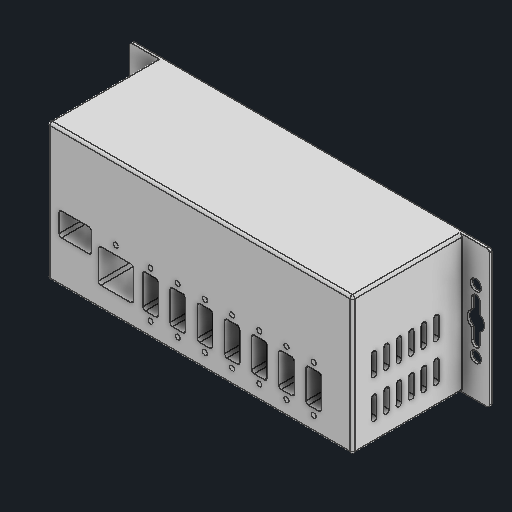
# Autodesk Inventor part: StarTech7PortUSB3Hub
Saved by Autodesk Inventor 2025.2 (Build 292293000, 293)
## iProperties
Created: 2025-10-31
Part Number: StarTech7PortUSB3Hub
Material: Generic
Document SubType Name: Modeling
Designer: valer
Density: 1 g/cm^3
Appearance: Default
Author: valer
Autodesk Inventor part; units mm, degrees
ref_plane "YZ Plane" through (0, 0, 0) normal (1, 0, 0) x (0, 1, 0)
ref_plane "XZ Plane" through (0, 0, 0) normal (0, 1, 0) x (-1, 0, 0)
ref_plane "XY Plane" through (0, 0, 0) normal (0, 0, 1) x (1, 0, 0)
sketch "Base" plane through (0, 0, 0) normal (0, 0, 1) x (1, 0, 0)
  line L0 (-72.25, -27.5) -> (72.25, -27.5)
  line L1 (72.25, -27.5) -> (72.25, 27.5)
  line L2 (72.25, 27.5) -> (-72.25, 27.5)
  line L3 (-72.25, 27.5) -> (-72.25, -27.5)
  line L4 (-72.25, -27.5) -> (72.25, 27.5) construction
  line L5 (72.25, -27.5) -> (-72.25, 27.5) construction
  line L6 (-66.75, 27.5) -> (-66.75, -27.5) construction
  line L7 (-101.15, 0) -> (101.15, 0) construction
  line L8 (0, -38.5) -> (0, 38.5) construction
  line L9 (66.75, 27.5) -> (66.75, -27.5) construction
  circle A0 centre (-66.75, 12.5) radius 2.25
  circle A1 centre (-66.75, -12.5) radius 2.25
  circle A2 centre (66.75, 12.5) radius 2.25
  circle A3 centre (66.75, -12.5) radius 2.25
  circle A4 centre (-66.75, 0) radius 3.5
  circle A5 centre (66.75, 0) radius 3.5
  circle A6 centre (-66.75, 7.5) radius 1.75
  circle A7 centre (-66.75, -7.5) radius 1.75
  line L10 (-68.5, 7.5) -> (-68.5, -7.5)
  line L11 (-65, 7.5) -> (-65, -7.5)
  circle A8 centre (66.75, 7.5) radius 1.75
  circle A9 centre (66.75, -7.5) radius 1.75
  line L12 (68.5, 7.5) -> (68.5, -7.5)
  line L13 (65, 7.5) -> (65, -7.5)
  point P0 (0, 0)
  point P1 (-65, -3.0311)
  point P2 (-68.5, -3.0311)
  point P3 (-68.5, 3.0311)
  point P4 (-65, 3.0311)
  point P5 (65, -3.0311)
  point P6 (65, 3.0311)
  point P7 (68.5, 3.0311)
  point P8 (68.5, -3.0311)
  dimension "d0" = 144.5
  dimension "d1" = 55
  dimension "d2" = 133.5
  dimension "d3" = 4.5
  dimension "d4" = 15
  dimension "d5" = 7
  dimension "d6" = 3.5
  dimension "d7" = 20
  constraints: 24 end point, 13 symmetric about line, 10 centre point, 8 point on circle, 5 point on line, 4 tangent, 3 midpoint, 2 parallel, 2 perpendicular, 1 horizontal, 7 other
  measures "d0" distance of L1.end L2.end
  measures "d1" distance of L0.end L1.end
  measures "d2" distance between parallel lines of L9 L6
  measures "d3" diameter of A0
  measures "d4" distance from line of L2 A0.centre
  measures "d5" diameter of A4
  measures "d6" diameter of A6
  measures "d7" distance of A1.centre A6.centre
extrude "BaseFeature" add sketch "Base" along normal blind 1
fillet "BaseFilletsFeature" radius 1 4 edges at (-72.25, -27.5, 0.5) (-72.25, 27.5, 0.5) (72.25, -27.5, 0.5) (72.25, 27.5, 0.5)
sketch "Sketch2" plane through (0, 0, 1) normal (0, 0, 1) x (1, 0, 0)
  line L0 (71.25, 27.5) -> (-71.25, 27.5) projected
  line L1 (-71.25, -27.5) -> (71.25, -27.5) projected
  line L2 (-61.25, 27.5) -> (61.25, 27.5)
  line L3 (61.25, 27.5) -> (61.25, -27.5)
  line L4 (61.25, -27.5) -> (-61.25, -27.5)
  line L5 (-61.25, -27.5) -> (-61.25, 27.5)
  line L6 (-72.25, 26.5) -> (-72.25, -26.5) projected
  line L7 (72.25, -26.5) -> (72.25, 26.5) projected
  point P0 (0, 0)
  point P1 (-61.25, -27.5)
  point P2 (61.25, 27.5)
  dimension "d11" = 11
  dimension "d12" = 11
  constraints: 8 end point, 2 parallel, 2 point on line, 1 horizontal, 1 perpendicular
  measures "d11" distance between parallel lines of L6 L5
  measures "d12" distance between parallel lines of L7 L3
extrude "BodyFeature" add sketch "Sketch2" along normal blind 44
fillet "BodyFilletsFeature" radius 1 4 edges at (-61.25, -27.5, 23) (-61.25, 27.5, 23) (61.25, -27.5, 23) (61.25, 27.5, 23)
sketch "Sketch3" plane through (0, 0, 45) normal (0, 0, 1) x (1, 0, 0)
  line L0 (-40.8, -1.85) -> (48.77, -1.85) construction
  line L1 (48.77, -1.85) -> (48.77, -22.35) construction
  line L2 (48.77, -22.35) -> (-40.8, -22.35) construction
  line L3 (-40.8, -22.35) -> (-40.8, -1.85) construction
  arc A0 (65, 3.0311) -> (65, -3.0311) centre (66.75, 0) ccw projected
  line L4 (48.77, -2.85) -> (-40.8, -2.85) construction
  line L5 (48.77, -12.1) -> (-40.8, -12.1) construction
  circle A1 centre (45.67, -2.85) radius 1
  line L6 (42.57, -5.35) -> (48.77, -5.35)
  line L7 (48.77, -5.35) -> (48.77, -18.85)
  line L8 (48.77, -18.85) -> (42.57, -18.85)
  line L9 (42.57, -18.85) -> (42.57, -5.35)
  line L10 (45.67, -2.85) -> (45.67, -12.1) construction
  circle A2 centre (45.67, -21.35) radius 1
  line L11 (61.25, -26.5) -> (61.25, 26.5) construction
  line L12 (31.65, -5.35) -> (37.85, -5.35)
  line L13 (31.65, -18.85) -> (31.65, -5.35)
  line L14 (37.85, -18.85) -> (31.65, -18.85)
  line L15 (37.85, -5.35) -> (37.85, -18.85)
  circle A3 centre (34.75, -2.85) radius 1
  circle A4 centre (34.75, -21.35) radius 1
  line L16 (20.73, -5.35) -> (26.93, -5.35)
  line L17 (20.73, -18.85) -> (20.73, -5.35)
  line L18 (26.93, -18.85) -> (20.73, -18.85)
  line L19 (26.93, -5.35) -> (26.93, -18.85)
  circle A5 centre (23.83, -2.85) radius 1
  circle A6 centre (23.83, -21.35) radius 1
  line L20 (9.81, -5.35) -> (16.01, -5.35)
  line L21 (9.81, -18.85) -> (9.81, -5.35)
  line L22 (16.01, -18.85) -> (9.81, -18.85)
  line L23 (16.01, -5.35) -> (16.01, -18.85)
  circle A7 centre (12.91, -2.85) radius 1
  circle A8 centre (12.91, -21.35) radius 1
  line L24 (-1.11, -5.35) -> (5.09, -5.35)
  line L25 (-1.11, -18.85) -> (-1.11, -5.35)
  line L26 (5.09, -18.85) -> (-1.11, -18.85)
  line L27 (5.09, -5.35) -> (5.09, -18.85)
  circle A9 centre (1.99, -2.85) radius 1
  circle A10 centre (1.99, -21.35) radius 1
  line L28 (-12.03, -5.35) -> (-5.83, -5.35)
  line L29 (-12.03, -18.85) -> (-12.03, -5.35)
  line L30 (-5.83, -18.85) -> (-12.03, -18.85)
  line L31 (-5.83, -5.35) -> (-5.83, -18.85)
  circle A11 centre (-8.93, -2.85) radius 1
  circle A12 centre (-8.93, -21.35) radius 1
  line L32 (-22.95, -5.35) -> (-16.75, -5.35)
  line L33 (-22.95, -18.85) -> (-22.95, -5.35)
  line L34 (-16.75, -18.85) -> (-22.95, -18.85)
  line L35 (-16.75, -5.35) -> (-16.75, -18.85)
  circle A13 centre (-19.85, -2.85) radius 1
  circle A14 centre (-19.85, -21.35) radius 1
  line L36 (-26.8, -5.35) -> (-40.8, -5.35)
  line L37 (-40.8, -5.35) -> (-40.8, -18.85)
  line L38 (-40.8, -18.85) -> (-26.8, -18.85)
  line L39 (-26.8, -18.85) -> (-26.8, -5.35)
  line L40 (-33.8, -2.85) -> (-33.8, -22.35) construction
  line L41 (-56.6, -0.85) -> (-43.6, -0.85)
  line L42 (-43.6, -0.85) -> (-43.6, -10.25)
  line L43 (-43.6, -10.25) -> (-56.6, -10.25)
  line L44 (-56.6, -10.25) -> (-56.6, -0.85)
  line L45 (-61.25, 26.5) -> (-61.25, -26.5) construction
  circle A15 centre (-33.8, -1.85) radius 1
  circle A16 centre (-33.8, -22.35) radius 1
  circle A17 centre (-45.1, -13.6) radius 1.5
  line L46 (-43.6, -10.25) -> (-43.6, -13.6) construction
  line L47 (-40.8, -12.1) -> (-45.1, -12.1) construction
  point P0 (0, 0)
  point P1 (42.57, -12.1)
  point P2 (45.67, -5.35)
  point P3 (34.75, -5.35)
  point P4 (31.65, -12.1)
  point P5 (23.83, -5.35)
  point P6 (20.73, -12.1)
  point P7 (12.91, -5.35)
  point P8 (9.81, -12.1)
  point P9 (1.99, -5.35)
  point P10 (-1.11, -12.1)
  point P11 (-8.93, -5.35)
  point P12 (-12.03, -12.1)
  point P13 (-19.85, -5.35)
  point P14 (-22.95, -12.1)
  point P15 (-33.8, -5.35)
  point P16 (-50.1, -10.25)
  point P17 (-26.8, -12.1)
  dimension "d16" = 12.1
  dimension "d17" = 2
  dimension "d18" = 13.5
  dimension "d19" = 6.2
  dimension "d20" = 18.5
  dimension "d21" = 12.48
  dimension "d24" = 10.92
  dimension "d29" = 14
  dimension "d30" = 13.95
  dimension "d31" = 16.3
  dimension "d32" = 9.4
  dimension "d33" = 11.15
  dimension "d34" = 1
  dimension "d35" = 13
  dimension "d36" = 3
  constraints: 92 end point, 17 centre point, 12 point on line, 9 parallel, 7 midpoint, 7 perpendicular, 5 horizontal, 4 collinear, 3 tangent, 2 equal radius, 2 point on circle, 1 coincident, 1 symmetric about line, 85 other
  measures "d16" vertical distance of A0.centre L5.start
  measures "d17" diameter of A1
  measures "d18" distance of L6.end L7.end
  measures "d19" distance between parallel lines of L9 L7
  measures "d20" distance from line of A2.centre L4
  measures "d21" distance between parallel lines of L11 L1
  measures "d24" distance of L6.start L12.start
  measures "d29" distance of L37.end L38.end
  measures "d30" distance from line of A14.centre L40
  measures "d31" distance from line of point (-50.1, -10.25) L40
  measures "d32" distance of L41.end L42.end
  measures "d33" distance from line of L45 point (-50.1, -10.25)
  measures "d34" distance between parallel lines of L0 L41
  measures "d35" distance of L42.end L43.end
  measures "d36" diameter of A17
extrude "PortsFeature" cut sketch "Sketch3" against normal blind 20 contours A1 | L6 L7 L8 L9 | A2 | L12 L15 L14 L13 | A3 | A4 | L16 L19 L18 L17 | A5 | A6 | L20 L23 L22 L21 | A7 | A8 | L24 L27 L26 L25 | A9 | A10 | L28 L31 L30 L29 | A11 | A12 | L32 L35 L34 L33 | A13 | A14 | L39 L38 L37 L36 | L41 L42 L43 L44 | A15
fillet "PortFilletsFeature" radius 1 36 edges at (48.77, -5.35, 35) (42.57, -5.35, 35) (42.57, -18.85, 35) (48.77, -18.85, 35) (37.85, -5.35, 35) (31.65, -5.35, 35) (31.65, -18.85, 35) (37.85, -18.85, 35) (26.93, -5.35, 35) (20.73, -5.35, 35) (20.73, -18.85, 35) (26.93, -18.85, 35) (16.01, -5.35, 35) (9.81, -5.35, 35) (9.81, -18.85, 35) (16.01, -18.85, 35) (5.09, -5.35, 35) (-1.11, -5.35, 35) (-1.11, -18.85, 35) (5.09, -18.85, 35) (-5.83, -5.35, 35) (-12.03, -5.35, 35) (-12.03, -18.85, 35) (-5.83, -18.85, 35) (-16.75, -5.35, 35) (-22.95, -5.35, 35) (-22.95, -18.85, 35) (-16.75, -18.85, 35) (-26.8, -5.35, 35) (-40.8, -5.35, 35) (-40.8, -18.85, 35) (-26.8, -18.85, 35) (-43.6, -0.85, 35) (-56.6, -0.85, 35) (-56.6, -10.25, 35) (-43.6, -10.25, 35)
fillet "OutsideFilletsFeature" radius 1 8 edges at (-60.9571, 27.2071, 45) (-61.25, 0, 45) (-60.9571, -27.2071, 45) (0, -27.5, 45) (60.9571, -27.2071, 45) (61.25, 0, 45) (60.9571, 27.2071, 45) (0, 27.5, 45)
sketch "Sketch4" plane through (61.25, -26.5, 1) normal (1, 0, 0) x (0, 0, -1)
  line L0 (-44, 7.65) -> (-24, 7.65) construction
  line L1 (-35.35, 7.65) -> (0, 7.65) construction
  line L2 (0, 7.65) -> (0, 15.65) construction
  line L3 (0, 15.65) -> (-35.35, 15.65) construction
  line L4 (-35.35, 15.65) -> (-35.35, 7.65) construction
  line L5 (-43, -1) -> (0, -1) projected
  line L6 (-44, 53) -> (-44, 0) projected
  line L7 (-35.35, 22.85) -> (-35.35, 14.85) construction
  line L8 (-35.35, 14.85) -> (0, 14.85) construction
  line L9 (0, 22.85) -> (-35.35, 22.85) construction
  line L10 (0, 14.85) -> (0, 22.85) construction
  line L11 (-35.35, 30.05) -> (-35.35, 22.05) construction
  line L12 (-35.35, 22.05) -> (0, 22.05) construction
  line L13 (0, 30.05) -> (-35.35, 30.05) construction
  line L14 (0, 22.05) -> (0, 30.05) construction
  line L15 (-35.35, 7.65) -> (-35.35, 14.85) construction
  line L16 (-34.25, 7.65) -> (-34.25, 14.85)
  line L17 (-36.45, 14.85) -> (-36.45, 7.65)
  arc A0 (-36.45, 7.65) -> (-34.25, 7.65) centre (-35.35, 7.65) ccw
  arc A1 (-34.25, 14.85) -> (-36.45, 14.85) centre (-35.35, 14.85) ccw
  line L18 (0, 0) -> (0, 53) projected
  line L19 (-35.35, 18.85) -> (0, 18.85) construction
  line L20 (-34.25, 30.05) -> (-34.25, 22.85)
  line L21 (-36.45, 22.85) -> (-36.45, 30.05)
  arc A2 (-34.25, 30.05) -> (-36.45, 30.05) centre (-35.35, 30.05) ccw
  arc A3 (-36.45, 22.85) -> (-34.25, 22.85) centre (-35.35, 22.85) ccw
  arc A4 (-31.45, 7.65) -> (-29.25, 7.65) centre (-30.35, 7.65) ccw
  line L22 (-31.45, 14.85) -> (-31.45, 7.65)
  line L23 (-29.25, 7.65) -> (-29.25, 14.85)
  arc A5 (-29.25, 14.85) -> (-31.45, 14.85) centre (-30.35, 14.85) ccw
  arc A6 (-31.45, 22.85) -> (-29.25, 22.85) centre (-30.35, 22.85) ccw
  line L24 (-31.45, 22.85) -> (-31.45, 30.05)
  line L25 (-29.25, 30.05) -> (-29.25, 22.85)
  arc A7 (-29.25, 30.05) -> (-31.45, 30.05) centre (-30.35, 30.05) ccw
  arc A8 (-26.45, 7.65) -> (-24.25, 7.65) centre (-25.35, 7.65) ccw
  line L26 (-26.45, 14.85) -> (-26.45, 7.65)
  line L27 (-24.25, 7.65) -> (-24.25, 14.85)
  arc A9 (-24.25, 14.85) -> (-26.45, 14.85) centre (-25.35, 14.85) ccw
  arc A10 (-26.45, 22.85) -> (-24.25, 22.85) centre (-25.35, 22.85) ccw
  line L28 (-26.45, 22.85) -> (-26.45, 30.05)
  line L29 (-24.25, 30.05) -> (-24.25, 22.85)
  arc A11 (-24.25, 30.05) -> (-26.45, 30.05) centre (-25.35, 30.05) ccw
  arc A12 (-21.45, 7.65) -> (-19.25, 7.65) centre (-20.35, 7.65) ccw
  line L30 (-21.45, 14.85) -> (-21.45, 7.65)
  line L31 (-19.25, 7.65) -> (-19.25, 14.85)
  arc A13 (-19.25, 14.85) -> (-21.45, 14.85) centre (-20.35, 14.85) ccw
  arc A14 (-21.45, 22.85) -> (-19.25, 22.85) centre (-20.35, 22.85) ccw
  line L32 (-21.45, 22.85) -> (-21.45, 30.05)
  line L33 (-19.25, 30.05) -> (-19.25, 22.85)
  arc A15 (-19.25, 30.05) -> (-21.45, 30.05) centre (-20.35, 30.05) ccw
  arc A16 (-16.45, 7.65) -> (-14.25, 7.65) centre (-15.35, 7.65) ccw
  line L34 (-16.45, 14.85) -> (-16.45, 7.65)
  line L35 (-14.25, 7.65) -> (-14.25, 14.85)
  arc A17 (-14.25, 14.85) -> (-16.45, 14.85) centre (-15.35, 14.85) ccw
  arc A18 (-16.45, 22.85) -> (-14.25, 22.85) centre (-15.35, 22.85) ccw
  line L36 (-16.45, 22.85) -> (-16.45, 30.05)
  line L37 (-14.25, 30.05) -> (-14.25, 22.85)
  arc A19 (-14.25, 30.05) -> (-16.45, 30.05) centre (-15.35, 30.05) ccw
  arc A20 (-11.45, 7.65) -> (-9.25, 7.65) centre (-10.35, 7.65) ccw
  line L38 (-11.45, 14.85) -> (-11.45, 7.65)
  line L39 (-9.25, 7.65) -> (-9.25, 14.85)
  arc A21 (-9.25, 14.85) -> (-11.45, 14.85) centre (-10.35, 14.85) ccw
  arc A22 (-11.45, 22.85) -> (-9.25, 22.85) centre (-10.35, 22.85) ccw
  line L40 (-11.45, 22.85) -> (-11.45, 30.05)
  line L41 (-9.25, 30.05) -> (-9.25, 22.85)
  arc A23 (-9.25, 30.05) -> (-11.45, 30.05) centre (-10.35, 30.05) ccw
  point P0 (1, 26.5)
  point P1 (-35.35, 11.25)
  dimension "d41" = 8.65
  dimension "d42" = 8.65
  dimension "d46" = 7.2
  dimension "d51" = 1.1
  dimension "d54" = 5
  dimension "d59" = 7.2
  dimension "d60" = 8
  constraints: 78 end point, 48 point on circle, 24 centre point, 5 symmetric about line, 4 tangent, 3 collinear, 3 parallel, 2 horizontal, 2 midpoint, 2 perpendicular, 2 point on line, 1 vertical, 117 other
  measures "d41" distance between parallel lines of L5 L0
  measures "d42" distance between parallel lines of L6 L4
  measures "d46" distance of L3.end L7.start
  measures "d51" radius of A1
  measures "d54" distance of L1.start A4.centre
  measures "d59" distance between parallel lines of L0 L8
  measures "d60" distance between parallel lines of L9 L8
extrude "Extrusion4" cut sketch "Sketch4" against normal blind 20
equation "\"d42\" = d41"
body "Solid1"
